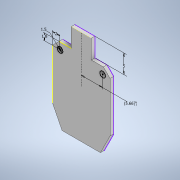
# Autodesk Inventor part: 1-3BT
Saved by Autodesk Inventor 2020 (Build 240168000, 168)
## iProperties
Created: 2019-10-01
Part Number: 1-3BT
Material: Generic
Document SubType Name: Modeling
Designer: yugio
Density: 1 g/cm^3
Appearance: Default
Author: yugio
Autodesk Inventor part; units mm, degrees
ref_plane "YZ Plane" through (0, 0, 0) normal (1, 0, 0) x (0, 1, 0)
ref_plane "XZ Plane" through (0, 0, 0) normal (0, 1, 0) x (-1, 0, 0)
ref_plane "XY Plane" through (0, 0, 0) normal (0, 0, 1) x (1, 0, 0)
sketch "Sketch1" plane through (0, 0, 0) normal (0, 0, 1) x (1, 0, 0)
  line L0 (76.6667, -74.52) -> (76.6667, 58.1502)
  line L1 (76.6667, 58.1502) -> (59.0237, 75.7932)
  line L2 (59.0237, 75.7932) -> (26.6667, 75.7932)
  line L3 (26.6667, 75.7932) -> (26.6667, 125.7932)
  line L4 (26.6667, 125.7932) -> (0, 125.7932)
  line L5 (0, 125.7932) -> (-26.6667, 125.7932)
  line L6 (-26.6667, 125.7932) -> (-26.6667, 75.7932)
  line L7 (-26.6667, 75.7932) -> (-59.0237, 75.7932)
  line L8 (-59.0237, 75.7932) -> (-76.6667, 58.1502)
  line L9 (-76.6667, 58.1502) -> (-76.6667, -74.52)
  line L10 (-76.6667, -74.52) -> (-51.0301, -125.7932)
  line L11 (-51.0301, -125.7932) -> (0, -125.7932)
  line L12 (0, -125.7932) -> (51.0301, -125.7932)
  line L13 (51.0301, -125.7932) -> (76.6667, -74.52)
  point P0 (0, 0)
  dimension "d0" = 50
  constraints: 28 end point, 2 perpendicular, 1 parallel
  measures "d0" distance of L3.start L4.start
extrude "Extrusion1" add sketch "Sketch1" along normal blind 9.525
sketch "Sketch2" plane through (0, 0, 9.525) normal (0, 0, 1) x (1, 0, 0)
  circle A0 centre (-56.6667, 57.7932) radius 7.5
  line L0 (0, 0) -> (0, 125.7932) construction
  line L1 (26.6667, 125.7932) -> (-26.6667, 125.7932) construction
  circle A1 centre (56.6667, 57.7932) radius 7.5
  line L2 (-26.6667, 75.7932) -> (-59.0237, 75.7932) projected
  line L3 (-76.6667, 58.1502) -> (-76.6667, -74.52) projected
  dimension "d3" = 18
  dimension "d4" = 20
  dimension "d5" = 15
  dimension "d8" = 56.6667
  constraints: 2 centre point, 2 end point, 1 midpoint, 1 symmetric about line, 1 other
  measures "d3" distance from line of L2 A0.centre
  measures "d4" distance from line of L3 A0.centre
  measures "d5" diameter of A0
  measures "d8" distance from line of L0 A1.centre
extrude "Extrusion2" cut sketch "Sketch2" against normal blind 9.525
body "Solid1"
